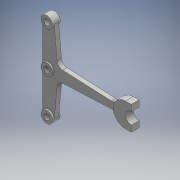
# Autodesk Inventor part: T di connessione1
Saved by Autodesk Inventor 2016 (Build 200138000, 138)
## iProperties
Created: 2016-12-04
Part Number: T di connessione1
Material: Generic
Document SubType Name: Modeling
Designer: Muhammad
Density: 1 g/cm^3
Appearance: Default
Author: Muhammad
Autodesk Inventor part; units mm, degrees
ref_plane "YZ Plane" through (0, 0, 0) normal (1, 0, 0) x (0, 1, 0)
ref_plane "XZ Plane" through (0, 0, 0) normal (0, 1, 0) x (-1, 0, 0)
ref_plane "XY Plane" through (0, 0, 0) normal (0, 0, 1) x (1, 0, 0)
sketch "Sketch1" plane through (0, 0, 0) normal (0, 1, 0) x (-1, 0, 0)
  circle A0 centre (0, 0) radius 6
  line L0 (6, 0) -> (6, -42.5)
  line L1 (6, 0) -> (6, 42.5)
  line L2 (6, 42.5) -> (0, 42.5) construction
  circle A1 centre (0, 42.5) radius 6
  circle A2 centre (0, -42.5) radius 6
  arc A3 (-5.9618, 43.1761) -> (6, 42.5) centre (0, 42.5) ccw
  line L3 (0, 42.5) -> (6, 42.5) construction
  line L4 (6, 0) -> (-13.7886, 0) construction
  line L5 (6, 0) -> (-10.1, 0) construction
  line L6 (0, 42.5) -> (-6, 42.4763) construction
  line L7 (-6, 42.4763) -> (-10.1, 0)
  line L8 (-6, -42.4763) -> (-10.1, 0)
  line L9 (-10.1, 0) -> (-9.499, 0) construction
  line L10 (-9.499, 0) -> (-9.5078, -6.135)
  line L11 (-9.499, 0) -> (-9.5078, 6.135)
  line L12 (0, 0) -> (-81.5, 0) construction
  line L13 (-69, 0) -> (-69, -3.393)
  line L14 (-69, -3.393) -> (-9.5078, -6.135)
  line L15 (-69, 0) -> (-69, 3.393)
  line L16 (-69, 3.393) -> (-9.5078, 6.135)
  point P0 (-69.4693, 3.393)
  dimension "d0" = 12
  dimension "d1" = 42.5
  dimension "d2" = 42.5
  dimension "d3" = 6
  dimension "d5" = 16.1
  dimension "d6" = 0.601
  dimension "d7" = 6.135
  dimension "d8" = 6.135
  dimension "d9" = 81.5
  constraints: 34 end point, 7 point on circle, 5 point on line, 4 vertical, 3 centre point, 3 coincident, 3 horizontal, 1 horizontal alignment, 1 perpendicular, 2 other
  measures "d1" distance of L0.start L0.end
  measures "d2" distance of L0.start L1.end
  measures "d3" distance of L1.end L2.end
  measures "d5" distance of L0.start L5.end
  measures "d6" distance of L5.end L9.end
  measures "d7" distance of L9.end L10.end
  measures "d8" distance of L9.end L11.end
  measures "d9" distance of L12.start L12.end
extrude "Extrusion1" add sketch "Sketch1" along normal mid plane 4.5 contours A0 | L0 A2 L8 L10 L11 L7 A1 L1 | A2 | A1 | L14 L13 L15 L16 L7 L8 | L8 L7 L11 L10
sketch "Sketch2" plane through (0, 0, 0) normal (0, 1, 0) x (-1, 0, 0)
  circle A0 centre (0, 0) radius 6
  line L0 (6, 0) -> (6, -42.5)
  line L1 (6, 0) -> (6, 42.5)
  line L2 (6, 42.5) -> (0, 42.5) construction
  circle A1 centre (0, 42.5) radius 6
  circle A2 centre (0, -42.5) radius 6
  arc A3 (-5.9618, 43.1761) -> (6, 42.5) centre (0, 42.5) ccw
  line L3 (0, 42.5) -> (6, 42.5) construction
  line L4 (6, 0) -> (-13.7886, 0) construction
  line L5 (6, 0) -> (-10.1, 0) construction
  line L6 (0, 42.5) -> (-6, 42.4763) construction
  line L7 (-6, 42.4763) -> (-10.1, 0)
  line L8 (-6, -42.4763) -> (-10.1, 0)
  line L9 (-10.1, 0) -> (-9.499, 0) construction
  line L10 (-9.499, 0) -> (-9.5078, -6.135)
  line L11 (-9.499, 0) -> (-9.5078, 6.135)
  line L12 (0, 0) -> (-81.5, 0) construction
  line L13 (-69, 0) -> (-69, -3.393)
  line L14 (-69, -3.393) -> (-9.5078, -6.135)
  line L15 (-69, 0) -> (-69, 3.393)
  line L16 (-69, 3.393) -> (-9.5078, 6.135)
  line L17 (-69, 0) -> (-81.5, 0)
  line L18 (-69, 3.393) -> (-69, -3.393) projected
  line L19 (-69, 3.393) -> (-69.4693, 3.393)
  line L20 (-69, -3.393) -> (-69.4693, -3.393)
  line L21 (-81.5, 12.5) -> (-87.5, 12.5)
  line L22 (-87.5, 12.5) -> (-87.5, -12.5)
  line L23 (-87.5, -12.5) -> (-81.5, -12.5)
  arc A4 (-81.5, -12.5) -> (-69.4693, -3.393) centre (-81.5, 0) ccw
  arc A5 (-69.4693, 3.393) -> (-81.5, 12.5) centre (-81.5, 0) ccw
  line L24 (-69, 3.393) -> (-69, -3.393)
  dimension "d19" = 12
  dimension "d20" = 42.5
  dimension "d21" = 42.5
  dimension "d22" = 6
  dimension "d23" = 16.1
  dimension "d24" = 0.601
  dimension "d25" = 6.135
  dimension "d26" = 6.135
  dimension "d27" = 81.5
  dimension "d28" = 12.5
  dimension "d29" = 6
  constraints: 48 end point, 12 point on circle, 6 horizontal, 5 centre point, 5 point on line, 5 vertical, 4 coincident, 2 perpendicular, 1 collinear, 1 horizontal alignment, 1 tangent, 2 other
  measures "d20" distance of L5.start L0.end
  measures "d21" distance of L5.start L1.end
  measures "d22" distance of L1.end L2.end
  measures "d23" distance of L5.start L9.start
  measures "d24" distance of L9.start L9.end
  measures "d25" distance of L9.end L10.end
  measures "d26" distance of L9.end L11.end
  measures "d27" distance of L12.start L12.end
  measures "d28" distance of L15.start L12.end
  measures "d29" distance of L21.start L21.end
extrude "Extrusion2" add sketch "Sketch2" along normal mid plane 8 contours A0 | A2 | A1 | L20 A4 L23 L22 L21 A5 L19 L15 L13
sketch "Sketch3" plane through (0, 4, 42.5) normal (0, 1, 0) x (1, 0, 0)
  circle A0 centre (0, 0) radius 3
  circle A1 centre (0, 42.5) radius 3
  arc A2 (-6, 85) -> (6, 84.9763) centre (0, 85) ccw projected
  circle A3 centre (0, 85) radius 3
  line L0 (87.5, 30) -> (87.5, 55) projected
  circle A4 centre (87.5, 42.5) radius 6
  dimension "d32" = 6
  dimension "d33" = 6
  dimension "d34" = 6
  dimension "d35" = 12
  constraints: 4 centre point, 2 coincident, 1 midpoint
  measures "d32" diameter of A0
  measures "d33" diameter of A1
  measures "d34" diameter of A3
  measures "d35" diameter of A4
extrude "Extrusion3" cut sketch "Sketch3" against normal through all
fillet "Fillet1" radius 6 4 edges at (69.4693, 0, 3.393) (69, 0, 3.393) (69, 0, -3.393) (69.4693, 0, -3.393)
fillet "Fillet2" radius 6 2 edges at (9.5078, 0, -6.135) (9.5078, 0, 6.135)
body "Solid1"
